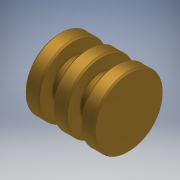
# Autodesk Inventor part: +XPanel_AntennaPost
Saved by Autodesk Inventor 2018 (Build 220112000, 112)
## iProperties
Created: 2018-10-28
Part Number: +XPanel_AntennaPost
Material: Brass, Soft Yellow
Document SubType Name: Modeling
Designer: Bradley
Density: 8.47 g/cm^3
Appearance: Brass - Satin
Mass: 0.583737 g
Surface Area: 1.64424 cm^2
Volume: 0.0689182 cm^3
Author: Bradley
Autodesk Inventor part; units mm, degrees
ref_plane "YZ Plane" through (0, 0, 0) normal (1, 0, 0) x (0, 1, 0)
ref_plane "XZ Plane" through (0, 0, 0) normal (0, 1, 0) x (-1, 0, 0)
ref_plane "XY Plane" through (0, 0, 0) normal (0, 0, 1) x (1, 0, 0)
sketch "Sketch1" plane through (0, 0, 0) normal (0, 1, 0) x (-1, 0, 0)
  line L0 (2.8, 0) -> (2.8, 1.5)
  line L1 (2.8, 1.5) -> (2.2, 1.5)
  line L2 (2.2, 1.5) -> (2.2, 2.5)
  line L3 (2.2, 2.5) -> (1.2, 2.5)
  line L4 (1.2, 2.5) -> (1.2, 1.5)
  line L5 (1.2, 1.5) -> (0.2, 1.5)
  line L6 (0.2, 1.5) -> (0.2, 2.5)
  line L7 (0.2, 2.5) -> (-0.8, 2.5)
  line L8 (-0.8, 2.5) -> (-0.8, 1.5)
  line L9 (-0.8, 1.5) -> (-1.8, 1.5)
  line L10 (-1.8, 1.5) -> (-1.8, 2.5)
  line L11 (-1.8, 2.5) -> (-2.8, 2.5)
  line L12 (-2.8, 2.5) -> (-2.8, 0)
  line L13 (-2.8, 0) -> (2.8, 0)
  point P0 (0, 0)
  point P1 (0, 0)
  dimension "d0" = 3
  dimension "d1" = 0.6
  dimension "d2" = 5
  dimension "d3" = 1
  dimension "d5" = 1
  dimension "d10" = 5.6
  constraints: 28 end point, 10 perpendicular, 6 point on line, 3 collinear, 1 coincident, 1 midpoint, 1 vertical
  measures "d0" diameter of L1 L13
  measures "d1" distance of L0.end L1.end
  measures "d2" diameter of L3 L13
  measures "d3" distance of L4.end L5.end
  measures "d5" distance of L3.end L4.end
  measures "d10" distance between parallel lines of L12 L0
revolve "Revolution1" add sketch "Sketch1" angle 360 about axis through (2.8, 0, 0) along (-1, 0, 0)
chamfer "Chamfer1" distance 0.1 angle 45 7 edges at (-2.2, 0, -2.5) (-1.2, 0, -2.5) (-0.2, 0, -2.5) (0.8, 0, -2.5) (1.8, 0, -2.5) (2.8, 0, -2.5) (-2.8, 0, -1.5)
body "Solid1"
